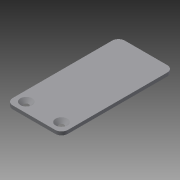
# Autodesk Inventor part: top v3
Saved by Autodesk Inventor 2014 (Build 180170000, 170)
## iProperties
Created: 2018-03-27
Part Number: top v3
Material: Generic
Document SubType Name: Modeling
Designer: HP820
Density: 1 g/cm^3
Appearance: Default
Author: HP820
Autodesk Inventor part; units mm, degrees
ref_plane "YZ Plane" through (0, 0, 0) normal (1, 0, 0) x (0, 1, 0)
ref_plane "XZ Plane" through (0, 0, 0) normal (0, 1, 0) x (-1, 0, 0)
sketch "Sketch1" plane through (0, 0, 0) normal (0, 0, 1) x (1, 0, 0)
  arc A0 (13.1, 23.6) -> (10.1, 26.6) centre (10.1, 23.6) ccw projected
  line L0 (10.1, 26.6) -> (-10.1, 26.6) projected
  arc A1 (-10.1, 26.6) -> (-13.1, 23.6) centre (-10.1, 23.6) ccw projected
  line L1 (-13.1, 23.6) -> (-13.1, -23.6) projected
  arc A2 (-13.1, -23.6) -> (-10.1, -26.6) centre (-10.1, -23.6) ccw projected
  line L2 (-10.1, -26.6) -> (10.1, -26.6) projected
  arc A3 (10.1, -26.6) -> (13.1, -23.6) centre (10.1, -23.6) ccw projected
  line L3 (13.1, -23.6) -> (13.1, 23.6) projected
  line L4 (11.5, 23) -> (11.5, -21.8566) projected
  line L5 (11.5, -21.8566) -> (11.5, -25) projected
  line L6 (11.5, -25) -> (8.3566, -25) projected
  line L7 (8.3566, -25) -> (-8.3566, -25) projected
  line L8 (-8.3566, -25) -> (-11.5, -25) projected
  line L9 (-11.5, -25) -> (-11.5, -21.8566) projected
  line L10 (-11.5, -21.8566) -> (-11.5, 23) projected
  line L11 (11.5, 23) -> (-11.5, 23) projected
  point P0 (0, 0)
extrude "Extrusion1" add sketch "Sketch1" along normal blind 1.6 contours L3 A3 L2 A2 L1 A1 L0 A0 | L4 L5 L6 L7 L8 L9 L10 L11
sketch "Sketch2" plane through (0, 0, 0) normal (0, 0, -1) x (-1, 0, 0)
  circle A0 centre (8.3566, -21.8566) radius 1.2 projected
  circle A1 centre (-8.3566, -21.8566) radius 1.2 projected
  point P0 (0, 0)
extrude "Extrusion2" cut sketch "Sketch2" against normal blind 1.6
chamfer "Chamfer1" distance 1.6 angle 45 2 edges at (9.5566, -21.8566, 1.6) (-7.1566, -21.8566, 1.6)
sketch "Sketch3" plane through (0, 0, 0) normal (0, 0, -1) x (-1, 0, 0)
  circle A0 centre (8.3566, -21.8566) radius 1.2 projected
  circle A1 centre (-8.3566, -21.8566) radius 1.2 projected
  arc A2 (-10.1, 26.6) -> (-13.1, 23.6) centre (-10.1, 23.6) ccw projected
  line L0 (-13.1, 23.6) -> (-13.1, -23.6) projected
  arc A3 (-13.1, -23.6) -> (-10.1, -26.6) centre (-10.1, -23.6) ccw projected
  line L1 (-10.1, -26.6) -> (10.1, -26.6) projected
  arc A4 (10.1, -26.6) -> (13.1, -23.6) centre (10.1, -23.6) ccw projected
  line L2 (13.1, -23.6) -> (13.1, 23.6) projected
  arc A5 (13.1, 23.6) -> (10.1, 26.6) centre (10.1, 23.6) ccw projected
  line L3 (10.1, 26.6) -> (-10.1, 26.6) projected
  point P0 (0, 0)
sketch "Sketch6" plane through (-13.1, -23.6, 1.6) normal (-1, 0, 0) x (0, 0, 1)
  line L0 (-1.6, 0) -> (-1.6, 47.2) projected
  line L1 (-1.6, 46.2477) -> (-2.136, 46.2477) projected
  line L2 (-2.136, 46.2477) -> (-3.0883, 47.2) projected
  line L3 (-3.0883, 47.2) -> (-3.0883, 48.4263) projected
  line L4 (-3.0883, 48.4263) -> (-3.8887, 48.4263) projected
  line L5 (-3.8887, 48.4263) -> (-3.8887, 44.7406) projected
  line L6 (-3.8887, 44.7406) -> (-1.6, 43.1845) projected
  line L7 (-1.6, 46.2477) -> (-1.6, 43.1845)
  point P0 (-1.6, 23.6)
  point P1 (-1.6, 1.7434)
  constraints: 2 end point, 1 collinear
extrude "Extrusion4" cut sketch "Sketch6" against normal blind 3
sketch "Sketch7" plane through (13.1, -23.6, 1.6) normal (1, 0, 0) x (0, 0, -1)
  line L0 (3.8887, 44.7406) -> (1.6, 43.1845) projected
  line L1 (3.8887, 48.4263) -> (3.8887, 44.7406) projected
  line L2 (3.0883, 48.4263) -> (3.8887, 48.4263) projected
  line L3 (3.0883, 47.2) -> (3.0883, 48.4263) projected
  line L4 (2.136, 46.2477) -> (3.0883, 47.2) projected
  line L5 (1.6, 46.2477) -> (2.136, 46.2477) projected
  line L6 (1.6, 46.2477) -> (1.6, 43.1845)
  point P0 (1.6, 23.6)
  constraints: 2 end point, 1 perpendicular
extrude "Extrusion5" cut sketch "Sketch7" against normal blind 3
ref_plane "Work Plane1" through (-10.1, -23.6, 0) normal (-1, 0, 0) x (0, 0, 1)
sketch "Sketch8" plane through (-10.1, -23.6, 0) normal (-1, 0, 0) x (0, 0, 1)
  line L0 (-0.536, 46.2477) -> (-1.4883, 47.2) projected
  line L1 (-1.4883, 47.2) -> (-1.4883, 48.4263) projected
  line L2 (-1.4883, 48.4263) -> (-2.2887, 48.4263) projected
  line L3 (-2.2887, 48.4263) -> (-2.2887, 44.7406) projected
  line L4 (-2.2887, 44.7406) -> (0, 43.1845) projected
  line L5 (0, 46.2477) -> (-0.536, 46.2477) projected
  line L6 (0, 0) -> (0, 47.2) projected
  point P0 (0, 23.6)
extrude "Extrusion6" add sketch "Sketch8" against normal blind 20
body "Solid1"
